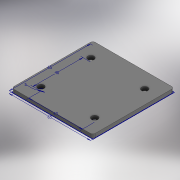
# Autodesk Inventor part: wheel_plate
Saved by Autodesk Inventor 2020 (Build 240168000, 168)
## iProperties
Created: 2020-06-18
Part Number: wheel_plate
Material: Generic
Document SubType Name: Modeling
Designer: pc-konvi
Density: 1 g/cm^3
Appearance: Gray
Author: pc-konvi
Autodesk Inventor part; units mm, degrees
ref_plane "YZ Plane" through (0, 0, 0) normal (1, 0, 0) x (0, 1, 0)
ref_plane "XZ Plane" through (0, 0, 0) normal (0, 1, 0) x (-1, 0, 0)
ref_plane "XY Plane" through (0, 0, 0) normal (0, 0, 1) x (1, 0, 0)
sketch "Sketch1" plane through (0, 0, 0) normal (0, 1, 0) x (-1, 0, 0)
  line L0 (-32.5, -32.5) -> (32.5, -32.5)
  line L1 (32.5, -32.5) -> (32.5, 32.5)
  line L2 (32.5, 32.5) -> (-32.5, 32.5)
  line L3 (-32.5, 32.5) -> (-32.5, -32.5)
  line L4 (-32.5, -32.5) -> (32.5, 32.5) construction
  line L5 (32.5, -32.5) -> (-32.5, 32.5) construction
  line L6 (-21.5, -20) -> (21.5, -20) construction
  line L7 (21.5, -20) -> (21.5, 20) construction
  line L8 (21.5, 20) -> (-21.5, 20) construction
  line L9 (-21.5, 20) -> (-21.5, -20) construction
  line L10 (-21.5, -20) -> (21.5, 20) construction
  line L11 (21.5, -20) -> (-21.5, 20) construction
  circle A0 centre (21.5, 20) radius 2.5
  point P0 (0, 0)
  dimension "d0" = 65
  dimension "d1" = 65
  dimension "d5" = 43
  dimension "d6" = 40
  dimension "d7" = 5
  constraints: 24 end point, 4 midpoint, 4 parallel, 2 horizontal, 2 perpendicular, 1 centre point, 1 coincident
  measures "d0" distance of L2.end L1.end
  measures "d1" distance of L1.end L0.end
  measures "d5" distance of L8.end L7.end
  measures "d6" distance of L7.end L6.end
  measures "d7" diameter of A0
extrude "Extrusion1" add sketch "Sketch1" along normal blind 3 contours L3 L2 L1 L0 | A0
fillet "Fillet1" radius 2 4 edges at (32.5, 1.5, 32.5) (32.5, 1.5, -32.5) (-32.5, 1.5, 32.5) (-32.5, 1.5, -32.5)
extrude "Extrusion2" cut sketch "Sketch1" along normal blind 3 contours A0
pattern_linear "Rectangular Pattern1" count 2 spacing 40 along (0, 0, -1) count 2 spacing 43 along (1, 0, 0) of "Extrusion2"
body "Solid1"
